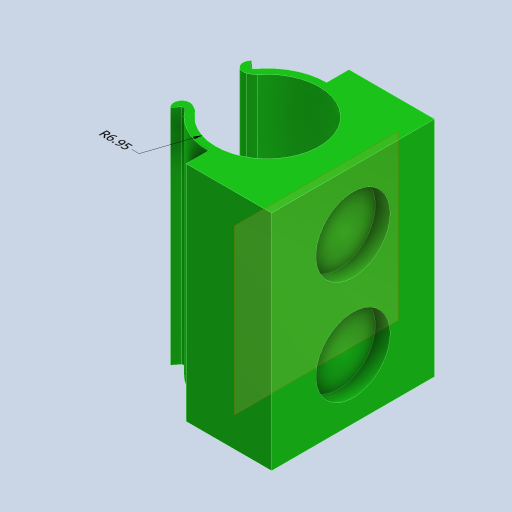
# Autodesk Inventor part: крепление маркера 14мм
Saved by Autodesk Inventor 2024.2 (Build 282272000, 272)
## iProperties
Created: 2025-12-12
Part Number: крепление маркера 14мм
Material: Типовые
Document SubType Name: Modeling
Designer: katya_notebook
Density: 1 g/cm^3
Appearance: Темно-зеленый
Author: katya_notebook
Autodesk Inventor part; units mm, degrees
ref_plane "YZ Plane" through (0, 0, 0) normal (1, 0, 0) x (0, 1, 0)
ref_plane "XZ Plane" through (0, 0, 0) normal (0, 1, 0) x (-1, 0, 0)
ref_plane "XY Plane" through (0, 0, 0) normal (0, 0, 1) x (1, 0, 0)
sketch "Эскиз1" plane through (0, 0, 0) normal (0, 1, 0) x (-1, 0, 0)
  circle A0 centre (0, 0) radius 6.95
  circle A1 centre (0, 0) radius 7.95
  line L0 (0, 0) -> (6.3439, 4.7913)
  line L1 (0, 0) -> (6.3439, -4.7913)
  point P0 (5.546, -4.1887)
  point P1 (5.546, 4.1887)
  dimension "d0" = 13.9
  dimension "d1" = 15.9
  constraints: 4 end point, 2 centre point, 2 coincident, 2 point on circle
  measures "d0" diameter of A0
  measures "d1" diameter of A1
extrude "Выдавливание1" add sketch "Эскиз1" along normal blind 30 contours A0 L1 A1 L0 picked at (-7.4629, 1.2262)
sketch "Эскиз2" plane through (0, 30, 0) normal (0, 1, 0) x (1, 0, 0)
  arc A0 (-5.546, -4.1887) -> (-6.4386, -3.6588) centre (-8.2473, -7.7226) ccw
  arc A1 (-6.4386, -3.6588) -> (-7.5956, -5.4645) centre (-6.873, -4.654) ccw
  line L0 (-7.5956, -5.4645) -> (-6.9243, -4.6101)
  arc A2 (-6.3454, -4.7768) -> (-6.9243, -4.6101) centre (-6.7137, -4.9672) ccw
  line L1 (-5.546, -4.1887) -> (-6.3439, -4.7913)
  line L2 (-6.3439, -4.7913) -> (-5.546, -4.1887)
  line L3 (-6.3439, -4.7913) -> (-6.3454, -4.7768)
  line L4 (-0.0151, 0) -> (-3.489, 0)
  arc A3 (-6.4386, 3.6588) -> (-5.546, 4.1887) centre (-8.2473, 7.7226) ccw
  arc A4 (-6.9243, 4.6101) -> (-6.3454, 4.7768) centre (-6.7137, 4.9672) ccw
  line L5 (-5.546, 4.1887) -> (-6.3439, 4.7913)
  line L6 (-6.3439, 4.7913) -> (-5.546, 4.1887)
  line L7 (-6.3439, 4.7913) -> (-6.3454, 4.7768)
  arc A5 (-7.5956, 5.4645) -> (-6.4386, 3.6588) centre (-6.873, 4.654) ccw
  line L8 (-7.5956, 5.4645) -> (-6.9243, 4.6101)
  point P0 (-5.546, 4.1887)
  point P1 (-6.3439, -4.7913)
  point P2 (-5.3694, -4.0591)
  point P3 (-6.3439, 4.7913)
  point P4 (-5.3694, 4.0591)
  point P5 (-6.3439, 4.7913)
  dimension "d25" = 1.0859
  constraints: 18 end point, 12 point on circle, 12 symmetric about line, 6 centre point, 4 coincident, 1 collinear, 1 horizontal, 3 other
  measures "d25" radius of A1
sketch "Эскиз3" plane through (0, 30, 0) normal (0, 1, 0) x (1, 0, 0)
  arc A0 (-6.3439, -4.7913) -> (-6.3439, 4.7913) centre (0, 0) ccw projected
  line L0 (11.5, -6.95) -> (11.5, 6.95)
  arc A1 (-5.546, -4.1887) -> (-5.546, 4.1887) centre (0, 0) ccw projected
  line L1 (0, -7.95) -> (0, -6.95)
  line L2 (0, 6.95) -> (0, 7.95)
  line L3 (11.5, 6.95) -> (11.5, 10.95)
  line L4 (11.5, -6.95) -> (11.5, -10.95)
  line L5 (0, 3.45) -> (0, 7.95)
  line L6 (11.5, -10.95) -> (0, -10.95)
  line L7 (0, -10.95) -> (0, -7.95)
  line L8 (11.5, 10.95) -> (0, 10.95)
  line L9 (0, 10.95) -> (0, 7.95)
  arc A2 (0, -6.95) -> (0, 6.95) centre (0, 0) ccw
  dimension "d13" = 4
  dimension "d14" = 4
  dimension "d22" = 21.9
  dimension "d23" = 4
  constraints: 20 end point, 6 point on circle, 4 vertical, 2 horizontal, 2 perpendicular, 1 centre point, 1 collinear, 1 concentric
  measures "d13" distance of L4.end L0.start
  measures "d14" distance of L3.end L0.end
  measures "d22" distance of L4.end L3.end
  measures "d23" distance of L6.end L1.end
extrude "Выдавливание3" add sketch "Эскиз3" against normal blind 30
ref_plane "РабПлоскость1" through (11.5, 20, 4.95) normal (1, 0, 0) x (0, 0, -1)
sketch "Эскиз4" plane through (11.5, 20, 4.95) normal (1, 0, 0) x (0, 0, -1)
  line L0 (4.95, -20) -> (4.95, 10)
  line L1 (1, 10) -> (8.9, 10) projected
  circle A0 centre (4.95, -12) radius 5
  line L2 (14.4, -20) -> (-4.5, -20) projected
  circle A1 centre (4.95, 2) radius 5
  line L3 (-4.5, 10) -> (14.4, 10) projected
  point P0 (7.3306, 10)
  point P1 (2.5694, 10)
  point P2 (4.95, 10)
  dimension "d15" = 10
  dimension "d16" = 8
  dimension "d17" = 10
  dimension "d18" = 8
  constraints: 3 midpoint, 2 centre point, 2 end point, 2 point on line
  measures "d15" diameter of A0
  measures "d16" distance of A0.centre point (4.95, -20)
  measures "d17" diameter of A1
  measures "d18" distance of point (4.95, 10) A1.centre
extrude "Выдавливание4" cut sketch "Эскиз4" against normal blind 2
extrude "Выдавливание5" add sketch "Эскиз2" against normal blind 30
sketch "Эскиз5" plane through (0, 30, 0) normal (0, 1, 0) x (1, 0, 0)
  arc A0 (0, 7.95) -> (-6.3439, 4.7913) centre (0, 0) ccw projected
  line L0 (-6.3439, 4.7913) -> (-6.3454, 4.7768) projected
  arc A1 (-6.9243, 4.6101) -> (-6.3454, 4.7768) centre (-6.7137, 4.9672) ccw projected
  line L1 (-6.9243, 4.6101) -> (-7.5956, 5.4645) projected
  arc A2 (-7.5956, 5.4645) -> (-6.4386, 3.6588) centre (-6.873, 4.654) ccw projected
  arc A3 (-6.4386, 3.6588) -> (-5.546, 4.1887) centre (-8.2473, 7.7226) ccw projected
  arc A4 (-5.546, -4.1887) -> (-5.546, 4.1887) centre (0, 0) ccw projected
  arc A5 (-5.546, -4.1887) -> (-6.4386, -3.6588) centre (-8.2473, -7.7226) ccw projected
  arc A6 (-6.4386, -3.6588) -> (-7.5956, -5.4645) centre (-6.873, -4.654) ccw projected
  line L2 (-7.5956, -5.4645) -> (-6.9243, -4.6101) projected
  arc A7 (-6.3454, -4.7768) -> (-6.9243, -4.6101) centre (-6.7137, -4.9672) ccw projected
  line L3 (-6.3454, -4.7768) -> (-6.3439, -4.7913) projected
  arc A8 (-6.3439, -4.7913) -> (0, -7.95) centre (0, 0) ccw projected
  line L4 (0, -7.95) -> (0, -10.95) projected
  line L5 (0, -10.95) -> (11.5, -10.95) projected
  line L6 (11.5, -10.95) -> (11.5, 10.95) projected
  line L7 (11.5, 10.95) -> (0, 10.95) projected
  line L8 (0, 10.95) -> (0, 7.95) projected
  line L9 (0, 6.95) -> (0, 7.95)
  line L10 (0, -6.95) -> (0, -7.95)
  constraints: 4 end point, 2 point on circle, 1 collinear, 1 point on line, 1 vertical
extrude "Выдавливание6" [suppressed]
sketch "Эскиз6" plane through (11.5, 30, 10.95) normal (1, 0, 0) x (0, 0, -1)
  arc A0 (15.95, -22) -> (15.95, -22) centre (10.95, -22) ccw projected
  arc A1 (15.95, -8) -> (15.95, -8) centre (10.95, -8) ccw projected
  point P0 (10.95, -30)
extrude "Выдавливание7" [suppressed]
